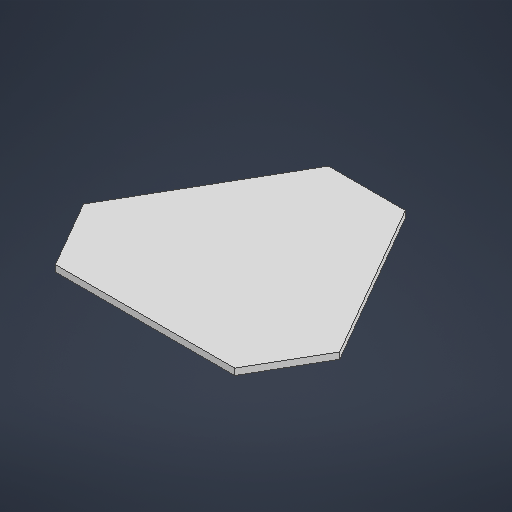
# Autodesk Inventor part: chassis
Saved by Autodesk Inventor 2026 (Build 300175000, 175)
## iProperties
Created: 2026-06-15
Part Number: chassis
Material: Generic
Document SubType Name: Modeling
Designer: Administrator
Density: 1 g/cm^3
Appearance: Default
Author: Administrator
Autodesk Inventor part; units mm, degrees
ref_plane "YZ Plane" through (0, 0, 0) normal (1, 0, 0) x (0, 1, 0)
ref_plane "XZ Plane" through (0, 0, 0) normal (0, 1, 0) x (-1, 0, 0)
ref_plane "XY Plane" through (0, 0, 0) normal (0, 0, 1) x (1, 0, 0)
sketch "Sketch1" plane through (0, 0, 0) normal (0, 1, 0) x (-1, 0, 0)
  line L0 (-18, -58.8877) -> (-59.9982, 13.8554)
  line L1 (-41.9982, 45.0323) -> (41.9982, 45.0323)
  line L2 (59.9982, 13.8554) -> (18, -58.8877)
  line L3 (41.9982, 45.0323) -> (59.9982, 13.8554)
  line L4 (18, -58.8877) -> (-18, -58.8877)
  line L5 (-41.9982, 45.0323) -> (-59.9982, 13.8554)
  point P0 (0, 0)
  point P1 (0, 0)
  dimension "d0" = 103.92
  dimension "d1" = 36
  dimension "d2" = 36
  dimension "d4" = 60
  dimension "d5" = 60
  dimension "d6" = 36
  dimension "d7" = 60
  constraints: 12 end point, 1 coincident, 4 other
  measures "d0" distance from line of L1 L2.end
  measures "d1" distance of L1.end L2.start
  measures "d2" distance of L2.end L0.start
  measures "d4" angle of L0 L4
  measures "d5" angle of L2 L3
  measures "d6" distance of L0.end L1.start
  measures "d7" angle of L1 L5
extrude "Extrusion1" add sketch "Sketch1" along normal blind 3
body "Solid1"
